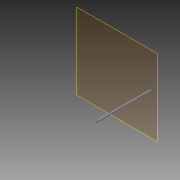
# Autodesk Inventor part: ArmCrossBrace
Saved by Autodesk Inventor 2013 (Build 170138000, 138)
## iProperties
Created: 2014-01-18
Part Number: ArmCrossBrace
Material: Generic
Document SubType Name: Modeling
Designer: 272817
Density: 1 g/cm^3
Author: 272817
Autodesk Inventor part; units mm, degrees
ref_plane "YZ Plane" through (0, 0, 0) normal (1, 0, 0) x (0, 1, 0)
ref_plane "XZ Plane" through (0, 0, 0) normal (0, 1, 0) x (-1, 0, 0)
ref_plane "XY Plane" through (0, 0, 0) normal (0, 0, 1) x (1, 0, 0)
ref_plane "Work Plane2" through (5.1191, 76.24, 0) normal (0, 0, 1) x (1, 0, 0)
sketch "Sketch1" plane through (5.1191, 76.24, 0) normal (0, 0, 1) x (1, 0, 0)
  circle A0 centre (-21.4407, 151.9494) radius 6.35
  point P0 (-5.1191, -76.24)
  dimension "d0" = 12.7
  constraints: 1 centre point
  measures "d0" diameter of A0
extrude "Extrusion1" add sketch "Sketch1" along normal blind 406.4
body "Solid1"
